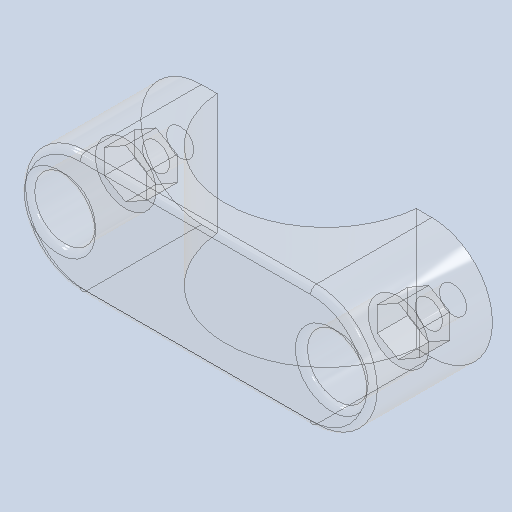
# Autodesk Inventor part: Uchwyt_silnika_2_dół
Saved by Autodesk Inventor 2023 (Build 270158000, 158)
## iProperties
Created: 2023-01-03
Part Number: Uchwyt_silnika_2_dół
Material: Tworzywo sztuczne PET
Document SubType Name: Modeling
Designer: komputer
Density: 1.541 g/cm^3
Appearance: Poliwęglan — przezroczysty
Author: komputer
Autodesk Inventor part; units mm, degrees
ref_plane "YZ Plane" through (0, 0, 0) normal (1, 0, 0) x (0, 1, 0)
ref_plane "XZ Plane" through (0, 0, 0) normal (0, 1, 0) x (-1, 0, 0)
ref_plane "XY Plane" through (0, 0, 0) normal (0, 0, 1) x (1, 0, 0)
sketch "Sketch1" plane through (0, 0, 0) normal (0, 0, 1) x (1, 0, 0)
  line L0 (19, 10) -> (-19, 10) projected
  arc A0 (19, -10) -> (19, 10) centre (19, 0) ccw projected
  line L1 (-19, -10) -> (19, -10) projected
  arc A1 (-19, 10) -> (-19, -10) centre (-19, 0) ccw projected
  circle A2 centre (22.5, 0) radius 2.25 projected
  circle A3 centre (-22.5, 0) radius 2.25 projected
  point P0 (0, 0)
extrude "Extrusion1" add sketch "Sketch1" along normal blind 20 contours A0 L1 A1 L0 | A2 | A3
sketch "Sketch2" plane through (-19, -10, 0) normal (0, -1, 0) x (1, 0, 0)
  arc A0 (3, 0) -> (35, 0) centre (19, 0) ccw projected
  line L0 (3, 0) -> (0, 0) projected
  line L1 (0, -40) -> (0, 0) projected
  line L2 (0, -40) -> (38, -40) projected
  line L3 (38, -40) -> (38, 0) projected
  line L4 (38, 0) -> (35, 0) projected
  circle A1 centre (19, 0) radius 16
  line L5 (0, 0) -> (38, 0) projected
  line L6 (38, 0) -> (38, 20) projected
  line L7 (0, 20) -> (38, 20) projected
  line L8 (0, 0) -> (0, 20) projected
  point P0 (19, 0)
  point P1 (3, 0)
  point P2 (35, 0)
  constraints: 1 centre point, 1 coincident, 1 concentric
extrude "Extrusion2" cut sketch "Sketch2" against normal through all contours A1 L5
sketch "Sketch3" plane through (0, 0, 20) normal (0, 0, 1) x (1, 0, 0)
  arc A0 (-19, 10) -> (-19, -10) centre (-19, 0) ccw projected
  line L0 (-19, -10) -> (19, -10) projected
  arc A1 (19, -10) -> (19, 10) centre (19, 0) ccw projected
  line L1 (19, 10) -> (-19, 10) projected
  line L2 (-16, -10.4231) -> (-16, -76.7035)
  arc A2 (-19, 10) -> (-19, -10) centre (-19, 0) ccw projected
  line L3 (-29, 0) -> (-16, 0)
  circle A3 centre (-22.5, 0) radius 2.25
  line L4 (19, 10) -> (-19, 10) projected
  line L5 (0, 10) -> (0, -10)
  circle A4 centre (22.5, 0) radius 2.25
  line L6 (-22.5, 0) -> (-26, 0)
  line L7 (-26, 2.0207) -> (-22.5, 4.0415)
  line L8 (-22.5, 4.0415) -> (-19, 2.0207)
  line L9 (-19, 2.0207) -> (-19, -2.0207)
  line L10 (-19, -2.0207) -> (-22.5, -4.0415)
  line L11 (-22.5, -4.0415) -> (-26, -2.0207)
  line L12 (-26, -2.0207) -> (-26, 2.0207)
  line L13 (26, 2.0207) -> (22.5, 4.0415)
  line L14 (22.5, 4.0415) -> (19, 2.0207)
  line L15 (19, 2.0207) -> (19, -2.0207)
  line L16 (19, -2.0207) -> (22.5, -4.0415)
  line L17 (22.5, -4.0415) -> (26, -2.0207)
  line L18 (26, -2.0207) -> (26, 2.0207)
  point P0 (0, 0)
  dimension "d4" = 4.5
  dimension "d5" = 3.5
  constraints: 32 end point, 7 symmetric about line, 4 midpoint, 2 centre point, 2 point on circle, 1 coincident, 1 horizontal, 1 point on line, 1 vertical, 16 other
  measures "d4" diameter of A3
  measures "d5" distance of L6.start L6.end
extrude "Extrusion3" [suppressed]
extrude "Extrusion4" cut sketch "Sketch3" against normal blind 5.5 contours L3 A3 | L3 A3 | A3 L3 L12 L7 L8 L9 | L3 L9 L10 L11 L12 A3 | A4 | L18 L17 L16 L15 L14 L13
extrude "Extrusion5" cut sketch "Sketch3" against normal through all contours L3 A3 | L3 A3 | A4
sketch "Sketch4" plane through (0, 0, 20) normal (0, 0, 1) x (1, 0, 0)
  line L0 (19, 2.0207) -> (22.5, 4.0415) projected
  line L1 (22.5, 4.0415) -> (26, 2.0207) projected
  line L2 (26, 2.0207) -> (26, -2.0207) projected
  line L3 (26, -2.0207) -> (22.5, -4.0415) projected
  line L4 (22.5, -4.0415) -> (19, -2.0207) projected
  line L5 (19, -2.0207) -> (19, 2.0207) projected
  line L6 (-19, -2.0207) -> (-22.5, -4.0415) projected
  line L7 (-22.5, -4.0415) -> (-26, -2.0207) projected
  line L8 (-26, -2.0207) -> (-26, 2.0207) projected
  line L9 (-26, 2.0207) -> (-22.5, 4.0415) projected
  line L10 (-22.5, 4.0415) -> (-19, 2.0207) projected
  line L11 (-19, 2.0207) -> (-19, -2.0207) projected
  arc A0 (-19, 10) -> (-19, -10) centre (-19, 0) ccw projected
  line L12 (-19, -10) -> (19, -10) projected
  arc A1 (19, -10) -> (19, 10) centre (19, 0) ccw projected
  line L13 (19, 10) -> (-19, 10) projected
  point P0 (0, 0)
extrude "Extrusion6" add sketch "Sketch4" along normal blind 1.5
sketch "Sketch5" plane through (0, 0, 0) normal (0, 0, -1) x (-1, 0, 0)
  circle A0 centre (-22.5, 0) radius 2.25 projected
  line L0 (-16, -10) -> (-16, 10) projected
  line L1 (-19, 10) -> (-16, 10) projected
  arc A1 (-19, 10) -> (-19, -10) centre (-19, 0) ccw projected
  line L2 (-16, -10) -> (-19, -10) projected
  circle A2 centre (22.5, 0) radius 2.25 projected
  line L3 (16, 10) -> (16, -10) projected
  line L4 (19, -10) -> (16, -10) projected
  arc A3 (19, -10) -> (19, 10) centre (19, 0) ccw projected
  line L5 (16, 10) -> (19, 10) projected
  point P0 (0, 0)
extrude "Extrusion7" cut sketch "Sketch5" against normal blind 0.5
sketch "Sketch6" plane through (0, -10, 0) normal (0, -1, 0) x (1, 0, 0)
  line L0 (-19, 0.5) -> (-19, 21.5) projected
  line L1 (-19, 0.5) -> (-16, 0.5) projected
  line L2 (-16, 0.5) -> (-16, 0) projected
  arc A0 (16, 0) -> (-16, 0) centre (0, 0) ccw projected
  line L3 (16, 0) -> (16, 0.5) projected
  line L4 (16, 0.5) -> (19, 0.5) projected
  line L5 (19, 0.5) -> (19, 21.5) projected
  arc A1 (16, 0) -> (-16, 0) centre (0, 0) ccw projected
  line L6 (0, 16) -> (0, 16.5)
  circle A2 centre (0, 0) radius 16.5
  line L7 (-19, 21.5) -> (19, 21.5) projected
  point P0 (0, 0)
  point P1 (16.4924, 0.5)
  point P2 (-16.4924, 0.5)
  dimension "d17" = 0.5
  constraints: 2 end point, 1 coincident, 1 point on circle, 1 vertical, 3 other
  measures "d17" distance of L6.start L6.end
extrude "Extrusion8" cut sketch "Sketch6" against normal through all contours A2 L6 A0 L2 L1 | A2 L4 L3 A0 L6
sketch "Sketch7" plane through (0, 0, 21.5) normal (0, 0, 1) x (1, 0, 0)
  circle A0 centre (-22.5, 0) radius 2.25 projected
  line L0 (-22.5, -4.0415) -> (-26, -2.0207) projected
  line L1 (-19, -2.0207) -> (-22.5, -4.0415) projected
  line L2 (-19, 2.0207) -> (-19, -2.0207) projected
  line L3 (-22.5, 4.0415) -> (-19, 2.0207) projected
  line L4 (-26, 2.0207) -> (-22.5, 4.0415) projected
  line L5 (-26, -2.0207) -> (-26, 2.0207) projected
  circle A1 centre (22.5, 0) radius 2.25 projected
  line L6 (22.5, 4.0415) -> (26, 2.0207) projected
  line L7 (19, 2.0207) -> (22.5, 4.0415) projected
  line L8 (19, -2.0207) -> (19, 2.0207) projected
  line L9 (22.5, -4.0415) -> (19, -2.0207) projected
  line L10 (26, -2.0207) -> (22.5, -4.0415) projected
  line L11 (26, 2.0207) -> (26, -2.0207) projected
  point P0 (0, 0)
extrude "Extrusion9" cut sketch "Sketch7" against normal blind 15
sketch "Sketch8" plane through (0, 0, 21.5) normal (0, 0, 1) x (1, 0, 0)
  line L0 (-19, -10) -> (19, -10) projected
  arc A0 (19, -10) -> (19, 10) centre (19, 0) ccw projected
  line L1 (19, 10) -> (-19, 10) projected
  arc A1 (-19, 10) -> (-19, -10) centre (-19, 0) ccw projected
  line L2 (-19, -2.0207) -> (-22.5, -4.0415) projected
  line L3 (-22.5, -4.0415) -> (-26, -2.0207) projected
  line L4 (-26, -2.0207) -> (-26, 2.0207) projected
  line L5 (-26, 2.0207) -> (-22.5, 4.0415) projected
  line L6 (-22.5, 4.0415) -> (-19, 2.0207) projected
  line L7 (-19, 2.0207) -> (-19, -2.0207) projected
  line L8 (19, 2.0207) -> (22.5, 4.0415) projected
  line L9 (22.5, 4.0415) -> (26, 2.0207) projected
  line L10 (26, 2.0207) -> (26, -2.0207) projected
  line L11 (26, -2.0207) -> (22.5, -4.0415) projected
  line L12 (22.5, -4.0415) -> (19, -2.0207) projected
  line L13 (19, -2.0207) -> (19, 2.0207) projected
  circle A2 centre (-22.5, 0) radius 2.25 projected
  circle A3 centre (22.5, 0) radius 2.25 projected
  circle A4 centre (-22.5, 0) radius 5
  circle A5 centre (22.5, 0) radius 5
  point P0 (0, 0)
  dimension "d22" = 10
  dimension "d23" = 10
  constraints: 2 centre point, 2 coincident
  measures "d22" diameter of A4
  measures "d23" diameter of A5
extrude "Extrusion10" cut sketch "Sketch8" against normal blind 11 contours L2 L3 L4 L5 L6 L7 | L8 L9 L10 L11 L12 L13 | A2 | A3 | A4 | A5
fillet "Fillet2" radius 1 6 edges at (0, -10, 21.5) (29, 0, 21.5) (0, 10, 21.5) (-29, 0, 21.5) (-27.5, 0, 21.5) (17.5, 0, 21.5)
sketch "Szkic9" plane through (0, 0, 6.5) normal (0, 0, 1) x (1, 0, 0)
  line L0 (-19, 2.0207) -> (-19, -2.0207) projected
  line L1 (-22.5, 4.0415) -> (-19, 2.0207) projected
  line L2 (-26, 2.0207) -> (-22.5, 4.0415) projected
  line L3 (-26, -2.0207) -> (-26, 2.0207) projected
  line L4 (-22.5, -4.0415) -> (-26, -2.0207) projected
  line L5 (-19, -2.0207) -> (-22.5, -4.0415) projected
  circle A0 centre (-22.5, 0) radius 2.25 projected
  line L6 (19, -2.0207) -> (19, 2.0207) projected
  line L7 (22.5, -4.0415) -> (19, -2.0207) projected
  line L8 (26, -2.0207) -> (22.5, -4.0415) projected
  line L9 (26, 2.0207) -> (26, -2.0207) projected
  line L10 (22.5, 4.0415) -> (26, 2.0207) projected
  line L11 (19, 2.0207) -> (22.5, 4.0415) projected
  circle A1 centre (22.5, 0) radius 2.25 projected
  point P0 (0, 0)
extrude "Wyciągnięcie proste11" cut sketch "Szkic9" against normal blind 1
sketch "Szkic10" plane through (0, 0, 0.5) normal (0, 0, -1) x (-1, 0, 0)
  line L0 (-16.4924, -10) -> (-16.4924, 10) projected
  line L1 (-19, 10) -> (-16.4924, 10) projected
  arc A0 (-19, 10) -> (-19, -10) centre (-19, 0) ccw projected
  line L2 (-16.4924, -10) -> (-19, -10) projected
  circle A1 centre (-22.5, 0) radius 2.25 projected
  circle A2 centre (22.5, 0) radius 2.25 projected
  line L3 (16.4924, 10) -> (16.4924, -10) projected
  line L4 (19, -10) -> (16.4924, -10) projected
  arc A3 (19, -10) -> (19, 10) centre (19, 0) ccw projected
  line L5 (16.4924, 10) -> (19, 10) projected
  point P0 (0, 0)
extrude "Wyciągnięcie proste12" cut sketch "Szkic10" against normal blind 1
sketch "Szkic11" plane through (-16.4924, -10, 0.5) normal (-1, 0, 0) x (0, 0, 1)
  line L0 (0, 20) -> (0, 0) projected
  line L1 (1, 0) -> (0, 0) projected
  line L2 (1, 0) -> (1, 20) projected
  line L3 (0, 20) -> (1, 20) projected
  point P0 (-0.5, 10)
extrude "Wyciągnięcie proste13" cut sketch "Szkic11" against normal through all
body "Solid1"
